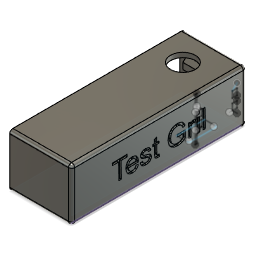
PacifierVape (Autodesk Fusion 360 design; units mm, degrees)
Autodesk Fusion 360 part; units mm, degrees
sketch "Side Profile" plane through (0, 0, 0) normal (0, 0, 1) x (1, 0, 0)
  line L0 (0, 0) -> (17, 0)
  line L1 (20, 3) -> (20, 14)
  line L2 (17, 17) -> (0, 17)
  line L3 (0, 17) -> (0, 0)
  line L4 (0, 0) -> (20, 0)
  line L5 (20, 0) -> (20, 17)
  line L6 (20, 17) -> (0, 17)
  line L7 (0, 17) -> (0, 0)
  point P0 (20, 0)
  point P1 (20, 17)
  dimension "d1" = 20
  dimension "d2" = 17
  constraint horizontal L0
  constraint vertical L1
  constraint horizontal L2
  constraint vertical L3
  constraint coincident L0.start L3.end
  constraint coincident P1 L1
  constraint coincident P1 L2
  constraint coincident P0 L0
  constraint coincident P0 L1
  constraint horizontal L4
  constraint vertical L5
  constraint horizontal L6
  constraint vertical L7
  constraint coincident P1 L5.end
  measures "d1" distance of L1 L3
  measures "d2" distance of P0 P1
extrude "Extrude1" add sketch "Side Profile" along normal blind 56.5
sketch "Button" plane through (0, 17, 0) normal (0, 1, 0) x (-1, 0, 0)
  line L0 (-20, 0) -> (0, 0)
  line L1 (0, 0) -> (0, 56.5)
  line L2 (0, 56.5) -> (-20, 56.5)
  circle A0 centre (-9, 9.5) radius 4
  line L3 (-20, 56.5) -> (-20, 0)
  dimension "d8" = 8
  dimension "d10" = 47
  measures "d8" diameter of A0
  measures "d10" distance of L2 A0.centre
shell "Shell1" thickness 1.5 removed faces 1 at (0, 11.3333, 18.8333)
extrude "Extrude2" cut sketch "Button" against normal blind 3 contours A0
fillet "Fillet1" radius 1 8 edges at (10, 17, 0) (20, 8.5, 0) (10, 0, 0) (20, 17, 28.25) (20, 0, 28.25) (20, 8.5, 56.5) (10, 17, 56.5) (10, 0, 56.5)
sketch "Text" plane through (20, 0, 0) normal (1, 0, 0) x (0, 0, -1)
  line L0 (-55.5, 16) -> (-55.5, 1)
  line L1 (-1, 1) -> (-1, 16)
  line L2 (-55.5, 1) -> (-0.7046, 2.1703) construction
  line L3 (-0.7046, 2.1703) -> (-1, 16) construction
  line L4 (-1, 16) -> (-55.7954, 14.8297) construction
  line L5 (-55.7954, 14.8297) -> (-55.5, 1) construction
  line L6 (-1, 16) -> (-55.5, 16)
  line L7 (-55.5, 1) -> (-1, 1)
  dimension "d16" = 6
  text T0 "Test Gril" font "Arial" height 6 align centre middle in box 54.8079 x 13.8328 at (-55.5, 1) x (0.999772, 0.021353) y (-0.021353, 0.999772) spacing 1 kerned
  constraint coincident L1.end
  constraint coincident L0.end
extrude "Extrude3" cut sketch "Text" against normal blind 0.5 text T0
sketch "USB" plane through (0, 0, 0) normal (0, -1, 0) x (1, 0, 0)
  line L0 (19, 55.5) -> (0, 55.5)
  line L1 (0, 55.5) -> (0, 1)
  line L2 (0, 1) -> (19, 1)
  line L3 (11.5, 5) -> (15, 5)
  line L4 (15.5, 5.5) -> (15.5, 13.5)
  line L5 (15, 14) -> (11.5, 14)
  line L6 (11.5, 14) -> (11.5, 5)
  arc A0 (15.5, 13.5) -> (15, 14) centre (15, 13.5) ccw
  arc A1 (15, 5) -> (15.5, 5.5) centre (15, 5.5) ccw
  line L7 (19, 1) -> (19, 55.5)
  dimension "d20" = 9
  dimension "d24" = 0.5
  dimension "d26" = 41.5
  dimension "d27" = 4
  constraint horizontal L3
  constraint vertical L4
  constraint horizontal L5
  constraint vertical L6
  constraint tangent L4 A0
  constraint tangent L5 A0
  constraint tangent L3 A1
  constraint tangent L4 A1
  constraint equal A0 A1
  measures "d20" distance of L3.start L5.end
  measures "d24" radius of A0
  measures "d26" distance of L0 L5
  measures "d27" distance of L4 L6
extrude "Extrude4" cut sketch "USB" against normal blind 3 contours L3 L4 L5 L6 A0 A1
sketch "Board Holder" plane through (18.5, 0, 0) normal (-1, 0, 0) x (0, 0, 1)
  line L0 (1.5, 15.5) -> (1.5, 1.5)
  line L1 (1.5, 1.5) -> (55, 1.5)
  line L2 (55, 1.5) -> (55, 15.5)
  line L3 (55, 15.5) -> (1.5, 15.5)
  line L4 (14.5, 15.5) -> (15, 15.5)
  line L5 (15, 15.5) -> (15, 1.5)
  line L6 (15, 1.5) -> (14.5, 1.5)
  line L7 (14.5, 1.5) -> (14.5, 15.5)
  line L8 (14.5, 8.5) -> (13, 8.5)
  line L9 (13, 8.5) -> (13, 10.5)
  line L10 (13, 10.5) -> (14.5, 10.5)
  line L11 (14.5, 10.5) -> (14.5, 8.5)
  line L12 (14.5, 12) -> (14.5, 11.5)
  line L13 (1.5, 8.5) -> (3, 8.5)
  line L14 (3, 8.5) -> (3, 10.5)
  line L15 (3, 10.5) -> (1.5, 10.5)
  line L16 (1.5, 10.5) -> (1.5, 8.5)
  line L17 (14.5, 7.5) -> (13, 7.5)
  line L18 (13, 7.5) -> (13, 5.5)
  line L19 (13, 5.5) -> (14.5, 5.5)
  line L20 (14.5, 5.5) -> (14.5, 7.5)
  line L21 (1.5, 7) -> (3, 7)
  line L22 (3, 7) -> (3, 5)
  line L23 (3, 5) -> (1.5, 5)
  line L24 (1.5, 5) -> (1.5, 7)
  line L25 (13, 10.5) -> (14.5, 12)
  line L26 (13, 10.5) -> (14.9142, 10.5) construction
  line L27 (13, 5.5) -> (14.5, 4)
  line L28 (13, 5.5) -> (14.9142, 5.5) construction
  line L29 (3, 10.5) -> (1.5, 12)
  line L30 (3, 5) -> (1.5, 3.5)
  line L31 (3, 5) -> (3.9142, 5) construction
  dimension "d39" = 0.5
  dimension "d40" = 40
  dimension "d41" = 1.5
  dimension "d42" = 2
  dimension "d43" = 7
  dimension "d48" = 7
  dimension "d52" = 1
  dimension "d53" = 1.5
  dimension "d56" = 45
  dimension "d57" = 45
  dimension "d58" = 135
  constraint horizontal L4
  constraint vertical L5
  constraint horizontal L6
  constraint vertical L7
  constraint coincident L1 L5.end
  constraint coincident L3 L4.start
  constraint horizontal L8
  constraint vertical L9
  constraint horizontal L10
  constraint vertical L11
  constraint coincident L7 L8.start
  constraint vertical L12
  constraint coincident L7 L12.end
  constraint horizontal L13
  constraint vertical L14
  constraint horizontal L15
  constraint vertical L16
  constraint coincident L0 L13.start
  constraint equal L9 L14
  constraint equal L8 L13
  constraint horizontal L17
  constraint vertical L18
  constraint horizontal L19
  constraint vertical L20
  constraint coincident L7 L17.start
  constraint equal L10 L17
  constraint equal L9 L18
  constraint horizontal L21
  constraint vertical L22
  constraint horizontal L23
  constraint vertical L24
  constraint coincident L0 L21.start
  constraint equal L10 L21
  constraint equal L9 L22
  constraint horizontal L26
  constraint coincident L7 L12.start
  constraint horizontal L28
  constraint coincident L7 L27.end
  constraint coincident L0 L29.end
  constraint horizontal L31
  constraint coincident L0 L30.end
  measures "d39" distance of L4.start L4.end
  measures "d40" distance of L2 L5
  measures "d41" distance of L9.end L10.end
  measures "d42" distance of L8.end L9.end
  measures "d43" distance of L1 L8
  measures "d48" distance of L1 L13
  measures "d52" distance of L8 L17
  measures "d53" distance of L13 L21
  measures "d56" angle of L25 L26
  measures "d57" angle of L27 L28
  measures "d58" angle of L30 L31
extrude "Extrude8" add sketch "Board Holder" along normal blind 16 contours L0 L15 L29 | L1 L3 L4 L5 L6 L7 L11 L12 L20 | L0 L13 L14 L15 L16 | L7 L10 L12 L25 | L7 L8 L9 L10 L11 | L0 L21 L22 L23 L24 | L0 L23 L30 | L7 L19 L27 | L7 L17 L18 L19 L20
equation "d2 = ShortSide"
equation "d43 = ( ShortSide / 2 ) - 1.5 mm"
equation "ShortSide = 17 mm"
equation "d48 = ( ShortSide / 2 ) - 1.5 mm"
named bodies: "Housing"
